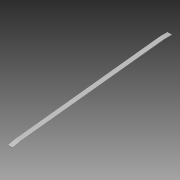
# Autodesk Inventor part: 2p6fs2
Saved by Autodesk Inventor 2014 (Build 180170000, 170)
## iProperties
Company: HERA Project
Created: 2013-12-11
Part Number: 2p6fs2
Material: Steel
Document SubType Name: Sheet Metal
Designer: David DeBoer
Mass: 1118.84 g
Surface Area: 1199.54 cm^2
Volume: 142.527 cm^3
Density: 7.85 g/cm^3
Description: second furring strip
Appearance: Steel
Sheet Metal Rule: Default
Author: David DeBoer
Autodesk Inventor part; units mm, degrees
ref_plane "YZ Plane" through (0, 0, 0) normal (1, 0, 0) x (0, 1, 0)
ref_plane "XZ Plane" through (0, 0, 0) normal (0, 1, 0) x (-1, 0, 0)
ref_plane "XY Plane" through (0, 0, 0) normal (0, 0, 1) x (1, 0, 0)
sketch "Sketch1" plane through (0, 0, 0) normal (0, 0, 1) x (1, 0, 0)
  line L0 (0, 0) -> (38.1, 0)
  line L1 (38.1, 0) -> (38.1, 3.048)
  line L2 (38.1, 3.048) -> (0, 3.048)
  line L3 (0, 3.048) -> (0, 0)
  dimension "d0" = 38.1
  dimension "d1" = 3.048
  constraints: 8 end point, 2 parallel, 1 horizontal, 1 perpendicular
  measures "d0" distance of L0.start L0.end
  measures "d1" distance of L2.end L0.start
extrude "Extrusion1" add sketch "Sketch1" along normal blind 1370
sketch "Sketch2" plane through (0, 3.048, 0) normal (0, 1, 0) x (1, 0, 0)
  line L0 (38.1, 0) -> (0, 0) projected
  circle A0 centre (19.05, -20) radius 2.2451
  dimension "d4" = 20
  constraints: 1 centre point
  measures "d4" distance from line of A0.centre L0
hole "Hole1" at (19.05, 3.048, 20) direction (0, -1, 0) diameter 3.175 end through all
sketch "Sketch3" plane through (0, 3.048, 0) normal (0, 1, 0) x (1, 0, 0)
  line L0 (38.1, -1370) -> (0, -1370) projected
  circle A0 centre (19.05, -1350) radius 2.2451
  dimension "d12" = 20
  constraints: 1 centre point
  measures "d12" distance from line of L0 A0.centre
hole "Hole2" at (19.05, 3.048, 1350) direction (0, -1, 0) diameter 3.175 end through all
sketch "Sketch4" plane through (0, 0, 0) normal (0, -1, 0) x (1, 0, 0)
  circle A0 centre (19.05, 20) radius 1.5875 projected
  line L0 (38.1, 0) -> (38.1, 1370) projected
  line L1 (0, 0) -> (0, 1370) projected
  line L2 (0, 60) -> (38.1, 60)
  line L3 (0, 60) -> (1.8993, 60)
  line L4 (0, 60) -> (38.1, 65.016)
  line L5 (0, 60) -> (38.1, 60) construction
  dimension "d20" = 40
  dimension "d21" = 7.5
  constraints: 8 end point, 4 point on line, 1 horizontal, 1 perpendicular
  measures "d20" distance from line of L2 A0.centre
  measures "d21" angle of L5 L4
fold "Fold1" angle 6.5 bend radius 3.048 thickness 3.048 k factor 0.44 line from (0, 0, 60) to (38.1, 0, 65.016) line at bend centre moving side (-0.1305262, 0, 0.9914449) folds toward (0, -1, 0)
sketch "Sketch6" plane through (0.02, -0.0196, 60.0995) normal (0.014776, -0.9935719, -0.1122347) x (0.9998905, 0.014776, 0.0008319)
  line L0 (38.1, 5.016) -> (38.1, 1309.7489) projected
  line L1 (0, 0) -> (0, 1309.7489) projected
  circle A0 centre (19.05, 1289.7489) radius 1.5875 projected
  line L2 (38.1, 1249.7489) -> (0, 1249.7489)
  line L3 (0, 1249.7489) -> (38.1, 1244.7329)
  line L4 (0, 1249.7489) -> (82.1613, 1249.7489) construction
  point P0 (-0.0697, -59.722)
  dimension "d35" = 40
  dimension "d36" = 7.5
  constraints: 6 end point, 3 point on line, 1 horizontal, 1 perpendicular
  measures "d35" distance from line of L2 A0.centre
  measures "d36" angle of L3 L4
fold "Fold3" angle 6.5 bend radius 3.048 thickness 3.048 k factor 0.44 line from (1.0596, -140.2848, 1301.9517) to (39.1512, -139.1589, 1296.9992) line at bend centre moving side (0.1313366, -0.1093459, 0.9852889) folds toward (0.014776, -0.9935719, -0.1122347)
equation "\"d1\" = Thickness"
equation "\"d22\" = BendReliefWidth"
equation "\"d23\" = BendReliefDepth"
equation "\"d24\" = MinimumRemnant"
equation "\"d25\" = BendRadius"
equation "\"d27\" = BendRadius"
equation "\"d37\" = BendReliefWidth"
equation "\"d38\" = BendReliefDepth"
equation "\"d39\" = MinimumRemnant"
equation "\"d40\" = BendRadius"
equation "\"d42\" = BendRadius"
equation "\"BendRadius\" = Thickness"
equation "\"BendReliefWidth\" = Thickness"
equation "\"BendReliefDepth\" = 0.5 * Thickness"
equation "\"CornerReliefSize\" = 4 * Thickness"
equation "\"MinimumRemnant\" = 2 * Thickness"
equation "\"TransitionRadius\" = BendRadius"
equation "\"JacobiRadiusSize\" = Thickness"
equation "\"GapSize\" = Thickness"
equation "\"Thickness\" = 3.048"
body "Solid1"
